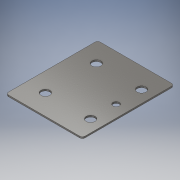
# Autodesk Inventor part: chapa-fixação-caixa-tubo
Saved by Autodesk Inventor 2019.4 (Build 234330000, 330)
## iProperties
Created: 2021-02-09
Part Number: chapa-fixação-caixa-tubo
Material: Aço galvanizado
Document SubType Name: Modeling
Designer: Lattes
Density: 7.85 g/cm^3
Appearance: Galvanizado
Author: Lattes
Autodesk Inventor part; units mm, degrees
ref_plane "YZ Plane" through (0, 0, 0) normal (1, 0, 0) x (0, 1, 0)
ref_plane "XZ Plane" through (0, 0, 0) normal (0, 1, 0) x (-1, 0, 0)
ref_plane "XY Plane" through (0, 0, 0) normal (0, 0, 1) x (1, 0, 0)
sketch "Esboço1" plane through (0, 0, 0) normal (0, 1, 0) x (-1, 0, 0)
  line L0 (0, 0) -> (60, 0)
  line L1 (60, 0) -> (60, -12)
  line L2 (60, -12) -> (60, -19)
  line L3 (60, -19) -> (60, -53)
  line L4 (60, -53) -> (60, -60)
  line L5 (60, -60) -> (60, -72)
  line L6 (60, -72) -> (0, -72)
  line L7 (0, -72) -> (0, 0)
  line L8 (0, 0) -> (19, 0)
  line L9 (60, 0) -> (30, 0)
  circle A0 centre (45, -16) radius 3.5
  circle A1 centre (45, -56) radius 3.5
  circle A2 centre (9.5, -16) radius 3.5
  circle A3 centre (9.5, -56) radius 3.5
  dimension "d0" = 60
  dimension "d1" = 12
  dimension "d2" = 7
  dimension "d3" = 34
  dimension "d4" = 7
  dimension "d5" = 12
  dimension "d6" = 72
  dimension "d7" = 19
  dimension "d12" = 30
  dimension "d23" = 7
  dimension "d24" = 7
  dimension "d25" = 7
  dimension "d26" = 7
  constraints: 20 end point, 4 centre point, 4 point on line, 3 perpendicular, 1 horizontal, 1 midpoint, 1 vertical
  measures "d0" distance of L0.start L0.end
  measures "d1" distance of L0.end L1.end
  measures "d2" distance of L1.end L2.end
  measures "d3" distance of L2.end L3.end
  measures "d4" distance of L3.end L4.end
  measures "d5" distance of L4.end L5.end
  measures "d6" distance of L6.end L0.start
  measures "d7" distance of L0.start L8.end
  measures "d12" distance of L0.end L9.end
  measures "d23" diameter of A0
  measures "d24" diameter of A1
  measures "d25" diameter of A2
  measures "d26" diameter of A3
extrude "Extrusão2" add sketch "Esboço1" along normal blind 1.2
fillet "Arredondamento2" radius 2 4 edges at (-60, 0.6, 0) (-60, 0.6, -72) (0, 0.6, 0) (0, 0.6, -72)
sketch "Esboço2" plane through (0, 1.2, 0) normal (0, 1, 0) x (1, 0, 0)
  circle A0 centre (-45, 56) radius 3.5 projected
  line L0 (-45, 56) -> (-30, 56)
  line L1 (-30, 56) -> (-20, 56)
  line L2 (0, 2) -> (0, 70) projected
  circle A1 centre (-9.5, 16) radius 3.5 projected
  circle A2 centre (-9.5, 36) radius 2.5
  point P0 (0, 0)
  dimension "d30" = 15
  dimension "d31" = 10
  dimension "d42" = 5
  constraints: 4 end point, 1 centre point, 1 horizontal, 1 point on line
  measures "d30" distance of L0.start L0.end
  measures "d31" distance of L0.end L1.end
  measures "d42" diameter of A2
extrude "Extrusão5" cut sketch "Esboço2" against normal blind 10 contours A2
